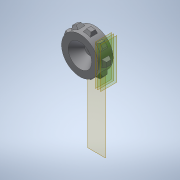
# Autodesk Inventor part: wheel
Saved by Autodesk Inventor 2020 (Build 240168000, 168)
## iProperties
Created: 2020-04-12
Part Number: wheel
Material: Ogólny
Document SubType Name: Modeling
Designer: blep
Density: 1 g/cm^3
Appearance: Domyślna
Author: blep
Autodesk Inventor part; units mm, degrees
ref_plane "YZ Plane" through (0, 0, 0) normal (1, 0, 0) x (0, 1, 0)
ref_plane "XZ Plane" through (0, 0, 0) normal (0, 1, 0) x (-1, 0, 0)
ref_plane "XY Plane" through (0, 0, 0) normal (0, 0, 1) x (1, 0, 0)
ref_plane "Płaszczyzna konstrukcyjna1" through (-6.2, -86.5, 1) normal (0, 0, 1) x (0, -1, 0)
sketch "Szkic1" plane through (-6.2, -86.5, 1) normal (0, 0, 1) x (0, -1, 0)
  arc A0 (-89.8717, 0.5902) -> (-95.3722, 1.2373) centre (-92, 6.2) ccw construction
  circle A1 centre (-92, 6.2) radius 10
  circle A2 centre (-92, 6.2) radius 25
  point P0 (-86.5, 6.2)
  dimension "d0" = 20
  dimension "d1" = 50
  constraints: 2 centre point, 2 coincident
  measures "d0" diameter of A1
  measures "d1" diameter of A2
extrude "Wyciągnięcie proste1" add sketch "Szkic1" along normal blind 20
ref_plane "Płaszczyzna konstrukcyjna2" through (0, 4.593, 6) normal (0, 0, 1) x (1, 0, 0)
sketch "Szkic3" plane through (0, 5.5, 21) normal (0, 0, 1) x (1, 0, 0)
  circle A0 centre (0, 0) radius 10 projected
  point P0 (0, -5.5)
extrude "Wyciągnięcie proste2" add sketch "Szkic3" against normal up to surface (20 mm away)
sketch "Szkic4" plane through (0, 5.5, 21) normal (0, 0, 1) x (1, 0, 0)
  circle A0 centre (0, 0) radius 25 construction
  circle A1 centre (0, 0) radius 2.25
  point P0 (0, -5.5)
  dimension "d6" = 4.5
  constraints: 1 centre point, 1 coincident
  measures "d6" diameter of A1
extrude "Wyciągnięcie proste3" cut sketch "Szkic4" against normal through all
ref_plane "Płaszczyzna konstrukcyjna4" through (25, 5.5, 1) normal (-1, 0, 0) x (0, -1, 0)
ref_plane "Płaszczyzna konstrukcyjna3" through (-8.2, -33.5, -38) normal (-1, 0, 0) x (0, 1, 0)
ref_plane "Płaszczyzna konstrukcyjna5" through (22, 5.5, 1) normal (-1, 0, 0) x (0, -1, 0)
sketch "Szkic5" plane through (22, 5.5, 1) normal (-1, 0, 0) x (0, -1, 0)
  line L0 (25, 0) -> (-25, 0) construction
  line L1 (25, 20) -> (-25, 20) construction
  line L2 (-25, 0) -> (-25, 20) construction
  line L3 (25, 0) -> (25, 20) construction
  line L4 (-6, 4) -> (6, 4)
  line L5 (6, 4) -> (6, 16)
  line L6 (6, 16) -> (-6, 16)
  line L7 (-6, 16) -> (-6, 4)
  line L8 (-6, 4) -> (-6, 0) construction
  line L9 (-6, 16) -> (-6, 20) construction
  line L10 (-6, 16) -> (-25, 16) construction
  line L11 (6, 16) -> (25, 16) construction
  point P0 (5.5, -1)
  dimension "d10" = 12
  dimension "d11" = 12
  constraints: 16 end point, 4 point on line, 3 horizontal, 2 collinear, 2 parallel, 2 vertical, 1 perpendicular
  measures "d10" distance of L4.end L5.end
  measures "d11" distance of L5.end L6.end
ref_plane "Płaszczyzna konstrukcyjna6" through (29, 5.5, 1) normal (-1, 0, 0) x (0, -1, 0)
sketch "Szkic6" plane through (29, 5.5, 1) normal (-1, 0, 0) x (0, -1, 0)
  line L0 (-6, 4) -> (6, 4) construction
  line L1 (6, 16) -> (-6, 16) construction
  line L2 (-6, 16) -> (-6, 4) construction
  line L3 (6, 4) -> (6, 16) construction
  line L4 (3, 7) -> (-3, 7)
  line L5 (-3, 7) -> (-3, 13)
  line L6 (-3, 13) -> (3, 13)
  line L7 (3, 13) -> (3, 7)
  point P0 (5.5, -1)
  dimension "d13" = 3
  constraints: 8 end point, 3 other
  measures "d13" distance between parallel lines of L0 L4
loft "Wyciągnięcie złożone1" add profiles "Szkic5", "Szkic6"
pattern_circular "Szyk kołowy1" count 9 over 360 about axis through (0, 5.5, 21) along (0, 0, -1) of "Wyciągnięcie złożone1"
sketch "Szkic8" plane through (0, 5.5, 1) normal (0, 0, -1) x (-1, 0, 0)
  circle A0 centre (0, 0) radius 2.25 projected
  circle A1 centre (0, 0) radius 25
  circle A2 centre (0, 0) radius 25 projected
  point P0 (0, -5.5)
  constraints: 1 centre point, 1 coincident, 1 concentric
extrude "Wyciągnięcie proste5" add sketch "Szkic8" along normal blind 7.6
sketch "Szkic10" plane through (0, 5.5, 21) normal (0, 0, 1) x (1, 0, 0)
  circle A0 centre (0, 0) radius 2.25 projected
  circle A1 centre (0, 0) radius 6
  point P0 (0, -5.5)
  dimension "d33" = 12
  constraints: 1 centre point, 1 coincident
  measures "d33" diameter of A1
sketch "Szkic11" plane through (0, 5.5, -6.6) normal (0, 0, -1) x (-1, 0, 0)
  circle A0 centre (0, 0) radius 8
  point P0 (0, -5.5)
  dimension "d36" = 16
  constraints: 1 centre point
  measures "d36" diameter of A0
extrude "Wyciągnięcie proste9" cut sketch "Szkic11" against normal blind 10
extrude "Wyciągnięcie proste10" cut sketch "Szkic10" against normal blind 12.6 contours A0 | A1
chamfer "Faza2" distance 10 distance2 12.6 1 edges at (-6, 5.5, 21)
sketch "Szkic15" plane through (0, 5.5, -6.6) normal (0, 0, -1) x (-1, 0, 0)
  arc A0 (7.9058, 5.3605) -> (9.21, 7.3062) centre (1.7819, 10.8751) ccw projected
  arc A1 (9.21, 7.3062) -> (8.6382, 7.974) centre (0, 0) ccw projected
  arc A2 (8.6382, 7.974) -> (6.5148, 6.9853) centre (11.0198, 0.0847) ccw projected
  arc A3 (6.5148, 6.9853) -> (5.9745, 7.4526) centre (0, 0) ccw projected
  arc A4 (5.9745, 7.4526) -> (6.6473, 9.6963) centre (-1.5027, 10.9172) ccw projected
  arc A5 (6.6473, 9.6963) -> (5.9041, 10.1659) centre (0, 0) ccw projected
  arc A6 (5.9041, 10.1659) -> (4.1664, 8.5952) centre (10.5053, 3.3291) ccw projected
  arc A7 (4.1664, 8.5952) -> (3.5124, 8.8825) centre (0, 0) ccw projected
  arc A8 (3.5124, 8.8825) -> (3.4939, 11.2248) centre (-4.6539, 9.9893) ccw projected
  arc A9 (3.4939, 11.2248) -> (2.6453, 11.4546) centre (0, 0) ccw projected
  arc A10 (2.6453, 11.4546) -> (1.4478, 9.4414) centre (9.0573, 6.2777) ccw projected
  arc A11 (1.4478, 9.4414) -> (0.7382, 9.5232) centre (0, 0) ccw projected
  arc A12 (0.7382, 9.5232) -> (0.0301, 11.756) centre (-7.3915, 8.1737) ccw projected
  arc A13 (0.0301, 11.756) -> (-0.8485, 11.7254) centre (0, 0) ccw projected
  arc A14 (-0.8485, 11.7254) -> (-1.3994, 9.4487) centre (6.8045, 8.6685) ccw projected
  arc A15 (-1.3994, 9.4487) -> (-2.1016, 9.3177) centre (0, 0) ccw projected
  arc A16 (-2.1016, 9.3177) -> (-3.4364, 11.2426) centre (-9.4724, 5.6319) ccw projected
  arc A17 (-3.4364, 11.2426) -> (-4.2669, 10.9544) centre (0, 0) ccw projected
  arc A18 (-4.2669, 10.9544) -> (-4.1223, 8.6164) centre (3.9471, 10.289) ccw projected
  arc A19 (-4.1223, 8.6164) -> (-4.7547, 8.2843) centre (0, 0) ccw projected
  arc A20 (-4.7547, 8.2843) -> (-6.5975, 9.7302) centre (-10.7116, 2.5897) ccw projected
  arc A21 (-6.5975, 9.7302) -> (-7.3062, 9.21) centre (0, 0) ccw projected
  arc A22 (-7.3062, 9.21) -> (-6.4789, 7.0186) centre (0.739, 10.9954) ccw projected
  arc A23 (-6.4789, 7.0186) -> (-6.9853, 6.5148) centre (0, 0) ccw projected
  arc A24 (-6.9853, 6.5148) -> (-9.1724, 7.3533) centre (-10.999, -0.6827) ccw projected
  arc A25 (-9.1724, 7.3533) -> (-9.6963, 6.6473) centre (0, 0) ccw projected
  arc A26 (-9.6963, 6.6473) -> (-8.2598, 4.7971) centre (-2.5347, 10.7247) ccw projected
  arc A27 (-8.2598, 4.7971) -> (-8.5952, 4.1664) centre (0, 0) ccw projected
  arc A28 (-8.5952, 4.1664) -> (-10.9323, 4.323) centre (-10.3091, -3.8944) ccw projected
  arc A29 (-10.9323, 4.323) -> (-11.2248, 3.4939) centre (0, 0) ccw projected
  arc A30 (-11.2248, 3.4939) -> (-9.3068, 2.1493) centre (-5.5833, 9.5011) ccw projected
  arc A31 (-9.3068, 2.1493) -> (-9.4414, 1.4478) centre (0, 0) ccw projected
  arc A32 (-9.4414, 1.4478) -> (-11.7209, 0.9086) centre (-8.7032, -6.76) ccw projected
  arc A33 (-11.7209, 0.9086) -> (-11.756, 0.0301) centre (0, 0) ccw projected
  arc A34 (-11.756, 0.0301) -> (-9.5268, -0.6894) centre (-8.1357, 7.4333) ccw projected
  arc A35 (-9.5268, -0.6894) -> (-9.4487, -1.3994) centre (0, 0) ccw projected
  arc A36 (-9.4487, -1.3994) -> (-11.468, -2.5866) centre (-6.324, -9.025) ccw projected
  arc A37 (-11.468, -2.5866) -> (-11.2426, -3.4364) centre (0, 0) ccw projected
  arc A38 (-11.2426, -3.4364) -> (-8.9004, -3.4669) centre (-9.9653, 4.705) ccw projected
  arc A39 (-8.9004, -3.4669) -> (-8.6164, -4.1223) centre (0, 0) ccw projected
  arc A40 (-8.6164, -4.1223) -> (-10.1961, -5.8519) centre (-3.3829, -10.4881) ccw projected
  arc A41 (-10.1961, -5.8519) -> (-9.7302, -6.5975) centre (0, 0) ccw projected
  arc A42 (-9.7302, -6.5975) -> (-7.4831, -5.9363) centre (-10.9094, 1.5587) ccw projected
  arc A43 (-7.4831, -5.9363) -> (-7.0186, -6.4789) centre (0, 0) ccw projected
  arc A44 (-7.0186, -6.4789) -> (-8.0182, -8.5973) centre (-0.1412, -11.0193) ccw projected
  arc A45 (-8.0182, -8.5973) -> (-7.3533, -9.1724) centre (0, 0) ccw projected
  arc A46 (-7.3533, -9.1724) -> (-5.4009, -7.8782) centre (-10.8841, -1.7262) ccw projected
  arc A47 (-5.4009, -7.8782) -> (-4.7971, -8.2598) centre (0, 0) ccw projected
  arc A48 (-4.7971, -8.2598) -> (-5.1279, -10.5787) centre (3.1131, -10.5713) ccw projected
  arc A49 (-5.1279, -10.5787) -> (-4.323, -10.9323) centre (0, 0) ccw projected
  arc A50 (-4.323, -10.9323) -> (-2.8388, -9.1202) centre (-9.8918, -4.8577) ccw projected
  arc A51 (-2.8388, -9.1202) -> (-2.1493, -9.3068) centre (0, 0) ccw projected
  arc A52 (-2.1493, -9.3068) -> (-1.7819, -11.6202) centre (6.0907, -9.1841) ccw projected
  arc A53 (-1.7819, -11.6202) -> (-0.9086, -11.7209) centre (0, 0) ccw projected
  arc A54 (-0.9086, -11.7209) -> (-0.0245, -9.5517) centre (-8.0205, -7.5575) ccw projected
  arc A55 (-0.0245, -9.5517) -> (0.6894, -9.5268) centre (0, 0) ccw projected
  arc A56 (0.6894, -9.5268) -> (1.7224, -11.6292) centre (8.5272, -6.9808) ccw projected
  arc A57 (1.7224, -11.6292) -> (2.5866, -11.468) centre (0, 0) ccw projected
  arc A58 (2.5866, -11.468) -> (2.792, -9.1346) centre (-5.4366, -9.5858) ccw projected
  arc A59 (2.792, -9.1346) -> (3.4669, -8.9004) centre (0, 0) ccw projected
  arc A60 (3.4669, -8.9004) -> (5.0736, -10.6049) centre (10.206, -4.1572) ccw projected
  arc A61 (5.0736, -10.6049) -> (5.8519, -10.1961) centre (0, 0) ccw projected
  arc A62 (5.8519, -10.1961) -> (5.3605, -7.9058) centre (-2.3696, -10.7624) ccw projected
  arc A63 (5.3605, -7.9058) -> (5.9363, -7.4831) centre (0, 0) ccw projected
  arc A64 (5.9363, -7.4831) -> (7.974, -8.6382) centre (10.9779, -0.9643) ccw projected
  arc A65 (7.974, -8.6382) -> (8.5973, -8.0182) centre (0, 0) ccw projected
  arc A66 (8.5973, -8.0182) -> (7.4526, -5.9745) centre (0.908, -10.9827) ccw projected
  arc A67 (7.4526, -5.9745) -> (7.8782, -5.4009) centre (0, 0) ccw projected
  arc A68 (7.8782, -5.4009) -> (10.1659, -5.9041) centre (10.7744, 2.3144) ccw projected
  arc A69 (10.1659, -5.9041) -> (10.5787, -5.1279) centre (0, 0) ccw projected
  arc A70 (10.5787, -5.1279) -> (8.8825, -3.5124) centre (4.1049, -10.2271) ccw projected
  arc A71 (8.8825, -3.5124) -> (9.1202, -2.8388) centre (0, 0) ccw projected
  arc A72 (9.1202, -2.8388) -> (11.4546, -2.6453) centre (9.6136, 5.3874) ccw projected
  arc A73 (11.4546, -2.6453) -> (11.6202, -1.7819) centre (0, 0) ccw projected
  arc A74 (11.6202, -1.7819) -> (9.5232, -0.7382) centre (6.937, -8.5628) ccw projected
  arc A75 (9.5232, -0.7382) -> (9.5517, -0.0245) centre (0, 0) ccw projected
  arc A76 (9.5517, -0.0245) -> (11.7254, 0.8485) centre (7.5985, 7.9817) ccw projected
  arc A77 (11.7254, 0.8485) -> (11.6292, 1.7224) centre (0, 0) ccw projected
  arc A78 (11.6292, 1.7224) -> (9.3177, 2.1016) centre (9.1527, -6.1377) ccw projected
  arc A79 (9.3177, 2.1016) -> (9.1346, 2.792) centre (0, 0) ccw projected
  arc A80 (9.1346, 2.792) -> (10.9544, 4.2669) centre (4.9083, 9.8668) ccw projected
  arc A81 (10.9544, 4.2669) -> (10.6049, 5.0736) centre (0, 0) ccw projected
  arc A82 (10.6049, 5.0736) -> (8.2843, 4.7547) centre (10.5552, -3.1672) ccw projected
  arc A83 (8.2843, 4.7547) -> (7.9058, 5.3605) centre (0, 0) ccw projected
  circle A84 centre (0, 0) radius 8 projected
  circle A85 centre (0, 0) radius 25 projected
  point P0 (0, -5.5)
extrude "Wyciągnięcie proste12" cut sketch "Szkic15" against normal blind 7.6 contours A85
